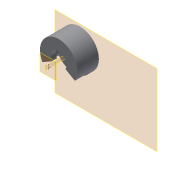
# Autodesk Inventor part: 101_Huawei_FilterLens_Adapter_Thread
Saved by Autodesk Inventor 2019 (Build 230136000, 136)
## iProperties
Created: 2019-06-17
Part Number: 101_Huawei_FilterLens_Adapter_Thread
Material: Generic
Document SubType Name: Modeling
Designer: diederichbenedict
Density: 1 g/cm^3
Appearance: Default
Author: diederichbenedict
Autodesk Inventor part; units mm, degrees
ref_plane "XZ Plane" through (0, 0, 0) normal (0, 1, 0) x (-1, 0, 0)
ref_plane "XY Plane" through (0, 0, 0) normal (0, 0, 1) x (1, 0, 0)
ref_plane "Work Plane1" through (0, 0, 0) normal (0, 0, 1) x (1, 0, 0)
ref_plane "Work Plane2" through (0, -6, 25.4) normal (0, 0, 1) x (1, 0, 0)
sketch "Sketch1" plane through (0, -6, 25.4) normal (0, 0, 1) x (1, 0, 0)
  point P0 (0, 6)
  point P1 (0, 6)
  constraints: 1 coincident
ref_plane "Work Plane3" through (0, 0, 25.4) normal (1, 0, 0) x (0, 1, 0)
sketch "Sketch2" plane through (0, 0, 25.4) normal (1, 0, 0) x (0, 1, 0)
  line L0 (12.6, -22.1) -> (12.6, -27.1) construction
  line L1 (8.75, -15.4) -> (8.75, -20.1) construction
  line L2 (-8.75, -15.4) -> (8.75, -15.4) construction
  arc A0 (-8.75, -20.1) -> (8.75, -20.1) centre (0, 0) ccw construction
  line L3 (-6, 0) -> (6, 0) construction
  line L4 (12.8, -25.4) -> (12.8, -21.9)
  line L5 (12.8, -21.9) -> (8.25, -21.9)
  line L6 (8.25, -21.9) -> (8.25, -20.6)
  line L7 (8.25, -20.6) -> (9.75, -20.6)
  line L8 (9.75, -20.6) -> (9.75, -15.0193)
  line L9 (9.75, -15.0193) -> (9.75, -12.4)
  line L10 (9.75, -12.4) -> (6.2, -12.4)
  line L11 (6.2, -12.4) -> (6.2, -8.4)
  line L12 (6.2, -8.4) -> (14.8, -8.4)
  line L13 (14.8, -8.4) -> (14.8, -25.4)
  line L14 (14.8, -25.4) -> (12.8, -25.4)
  line L15 (6, 0) -> (6, -15.4)
  line L16 (0, 0) -> (0, -25.4)
  dimension "d0" = 1
  dimension "d1" = 0.2
  dimension "d2" = 0.2
  dimension "d3" = 2
  dimension "d4" = 0.5
  dimension "d5" = 0.5
  dimension "d6" = 3
  dimension "d7" = 0.2
  dimension "d8" = 4
  constraints: 30 end point, 9 perpendicular, 5 vertical, 2 point on circle, 1 centre point, 1 point on line, 8 other
  measures "d0" distance between parallel lines of L1 L8
  measures "d1" distance between parallel lines of L0 L4
  measures "d2" distance from line of L0.start L5
  measures "d3" distance between parallel lines of L4 L13
  measures "d4" horizontal distance of L1.end L6.end
  measures "d5" horizontal distance of L6.end L1.end
  measures "d6" distance between parallel lines of L2 L10
  measures "d7" distance between parallel lines of L15 L11
  measures "d8" distance between parallel lines of L10 L12
revolve "Revolution1" add sketch "Sketch2" angle 240 mid plane about axis through (0, 0, 25.4) along (0, -0.0000003, -1)
sketch "Sketch3" plane through (-12.8172, -7.4, 0) normal (0.5, -0.8660254, 0.0000002) x (0.8660254, 0.5, -0.0000004)
  line L0 (2, 0) -> (2, 3.5) projected
  line L1 (2, 3.5) -> (6.55, 3.5) projected
  line L2 (6.55, 3.5) -> (6.55, 4.8) projected
  line L3 (6.55, 4.8) -> (5.05, 4.8) projected
  line L4 (5.05, 4.8) -> (5.05, 13) projected
  line L5 (5.05, 13) -> (8.6, 13) projected
  line L6 (8.6, 13) -> (8.6, 17) projected
  line L7 (8.6, 17) -> (0, 17) projected
  line L8 (0, 17) -> (0, 0) projected
  line L9 (0, 0) -> (2, 0) projected
  line L10 (5.05, 4.8) -> (5.05, 13) projected
  line L11 (5.05, 4.8) -> (0, 4.8)
  line L12 (14.8, -5.08) -> (14.8, 30.48) projected
  point P0 (14.8, 0)
  constraints: 2 end point, 1 perpendicular, 1 point on line
revolve "Revolution2" add sketch "Sketch3" angle 360 about axis through (0, 0, -10) along (-0.0000001, 0.0000002, 1) contours L9 L8 L11 L3 L2 L1 L0
body "Solid1"
